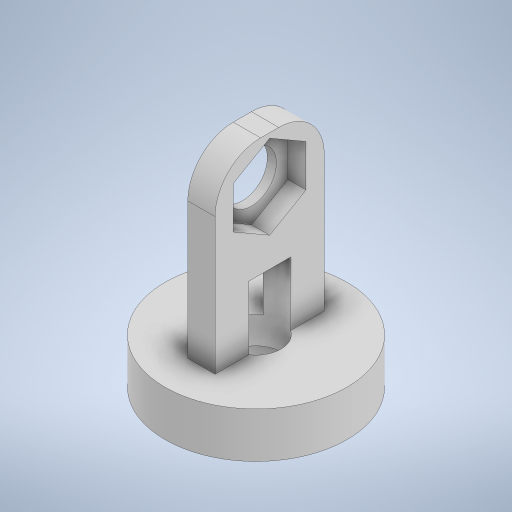
# Autodesk Inventor part: J2
Saved by Autodesk Inventor 2023 (Build 270158000, 158)
## iProperties
Created: 2023-12-18
Part Number: J2
Material: Generic
Document SubType Name: Modeling
Designer: Mustapha
Density: 1 g/cm^3
Appearance: Default
Author: Mustapha
Autodesk Inventor part; units mm, degrees
ref_plane "YZ Plane" through (0, 0, 0) normal (1, 0, 0) x (0, 1, 0)
ref_plane "XZ Plane" through (0, 0, 0) normal (0, 1, 0) x (-1, 0, 0)
ref_plane "XY Plane" through (0, 0, 0) normal (0, 0, 1) x (1, 0, 0)
sketch "Sketch1" plane through (0, 0, 0) normal (0, 1, 0) x (-1, 0, 0)
  line L0 (-10, 10) -> (10, 10)
  line L1 (10, 10) -> (10, -10)
  line L2 (10, -10) -> (-10, -10)
  line L3 (-10, -10) -> (-10, 10)
  line L4 (-10, 10) -> (10, -10) construction
  line L5 (10, 10) -> (-10, -10) construction
  point P0 (0, 0)
  dimension "d0" = 20
  dimension "d1" = 20
  constraints: 12 end point, 2 midpoint, 2 parallel, 1 horizontal, 1 perpendicular
  measures "d0" distance between parallel lines of L3 L1
  measures "d1" distance of L0.end L1.end
extrude "Extrusion1" add sketch "Sketch1" along normal blind 5
sketch "Sketch3" plane through (0, 0, 0) normal (0, -1, 0) x (1, 0, 0)
  line L0 (0, 4.6188) -> (4, 2.3094)
  line L1 (4, 2.3094) -> (4, -2.3094)
  line L2 (4, -2.3094) -> (0, -4.6188)
  line L3 (0, -4.6188) -> (-4, -2.3094)
  line L4 (-4, -2.3094) -> (-4, 2.3094)
  line L5 (-4, 2.3094) -> (0, 4.6188)
  line L6 (10, 10) -> (10, -10) projected
  point P0 (0, 0)
  point P1 (0, 0)
  point P2 (-4, 0)
  dimension "d7" = 8
  constraints: 12 end point, 1 coincident, 1 midpoint, 1 parallel, 13 other
  measures "d7" distance from line of L1 point (-4, 0)
extrude "Extrusion3" cut sketch "Sketch3" against normal blind 2
sketch "Sketch2" plane through (0, 0, 0) normal (0, -1, 0) x (1, 0, 0)
  circle A0 centre (0, 0) radius 2.75
  dimension "d4" = 5.5
  constraints: 1 centre point, 1 coincident
  measures "d4" diameter of A0
extrude "Extrusion2" cut sketch "Sketch2" against normal blind 22.5
sketch "Sketch4" plane through (0, 5, 0) normal (0, 1, 0) x (1, 0, 0)
  line L0 (1.5, 6) -> (-1.5, 6)
  line L1 (-1.5, 6) -> (-1.5, -6)
  line L2 (-1.5, -6) -> (1.5, -6)
  line L3 (1.5, -6) -> (1.5, 6)
  circle A0 centre (0, 0) radius 2.75 projected
  line L4 (1.5, 6) -> (-1.5, -6) construction
  line L5 (-1.5, 6) -> (1.5, -6) construction
  dimension "d10" = 6
  dimension "d11" = 3
  constraints: 12 end point, 2 midpoint, 2 parallel, 1 horizontal, 1 perpendicular
  measures "d10" distance from line of point (0, 0) L0
  measures "d11" distance between parallel lines of L1 L3
extrude "Extrusion4" add sketch "Sketch4" along normal blind 20 contours L3 A0 L1 L0 | L3 A0 L1 | L3 L2 L1 A0
sketch "Sketch5" plane through (0, 2, 0) normal (0, -1, 0) x (1, 0, 0)
  circle A0 centre (0, 0) radius 2.75
  dimension "d14" = 5.5
  constraints: 1 centre point, 1 coincident
  measures "d14" diameter of A0
extrude "Extrusion5" cut sketch "Sketch5" against normal blind 10
fillet "Fillet1" radius 10 4 edges at (-10, 2.5, -10) (-10, 2.5, 10) (10, 2.5, -10) (10, 2.5, 10)
fillet "Fillet2" radius 5 2 edges at (0, 25, -6) (0, 25, 6)
sketch "Sketch6" plane through (1.5, 5, 6) normal (1, 0, 0) x (0, 0, -1)
  line L0 (6, 19.4737) -> (10, 17.1643)
  line L1 (10, 17.1643) -> (10, 12.5455)
  line L2 (10, 12.5455) -> (6, 10.2361)
  line L3 (6, 10.2361) -> (2, 12.5455)
  line L4 (2, 12.5455) -> (2, 17.1643)
  line L5 (2, 17.1643) -> (6, 19.4737)
  line L6 (12, 0) -> (12, 15) projected
  point P0 (6, -5)
  point P1 (6, 14.8549)
  dimension "d21" = 8
  constraints: 12 end point, 1 parallel, 13 other
  measures "d21" distance between parallel lines of L4 L1
extrude "Extrusion6" cut sketch "Sketch6" against normal blind 2
sketch "Sketch7" plane through (-0.5, 5, 6) normal (1, 0, 0) x (0, 0, -1)
  circle A0 centre (6, 14.75) radius 2.75
  line L0 (12, 0) -> (12, 15) projected
  line L1 (5, 20) -> (7, 20) projected
  point P0 (6, -5)
  point P1 (6, 20)
  dimension "d24" = 5.5
  dimension "d25" = 6
  dimension "d26" = 5.25
  constraints: 1 centre point, 1 midpoint
  measures "d24" diameter of A0
  measures "d25" distance from line of L0 A0.centre
  measures "d26" distance of point (6, 20) A0.centre
extrude "Extrusion7" cut sketch "Sketch7" against normal blind 40.5
body "Solid1"
